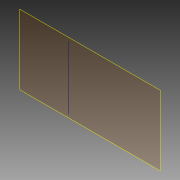
# Autodesk Inventor part: BlueLineMarking
Saved by Autodesk Inventor 2013 (Build 170138000, 138)
## iProperties
Created: 2013-01-07
Part Number: BlueLineMarking
Material: ABS Plastic
Document SubType Name: Modeling
Designer: Phillip
Density: 1 g/cm^3
Author: Phillip
Autodesk Inventor part; units mm, degrees
ref_plane "YZ Plane" through (0, 0, 0) normal (1, 0, 0) x (0, 1, 0)
ref_plane "XZ Plane" through (0, 0, 0) normal (0, 1, 0) x (-1, 0, 0)
ref_plane "XY Plane" through (0, 0, 0) normal (0, 0, 1) x (1, 0, 0)
ref_plane "Work Plane1" through (0, 0, 0) normal (0, 0, 1) x (1, 0, 0)
sketch "Sketch1" plane through (0, 0, 0) normal (0, 0, 1) x (1, 0, 0)
  line L0 (-2770.9482, 4082.669) -> (-2720.1482, 4082.669)
  line L1 (-2720.1482, 4082.669) -> (-2720.1482, -4082.669)
  line L2 (-2720.1482, -4082.669) -> (-2770.9482, -4082.669)
  line L3 (-2770.9482, -4082.669) -> (-2770.9482, 4082.669)
  line L4 (-8248.396, -4082.669) -> (8248.396, -4082.669) projected
  line L5 (8248.396, -4082.669) -> (8248.396, 4082.669) projected
  line L6 (8248.396, 4082.669) -> (-8248.396, 4082.669) projected
  line L7 (-8248.396, 4082.669) -> (-8248.396, -4082.669) projected
  point P0 (0, 0)
  dimension "d0" = 50.8
  constraints: 8 end point, 2 collinear, 2 parallel, 1 horizontal, 1 perpendicular
  measures "d0" distance of L0.start L0.end
extrude "Extrusion1" add sketch "Sketch1" along normal blind 2.54 contours L0 L1 L2 L3
body "Solid1"
